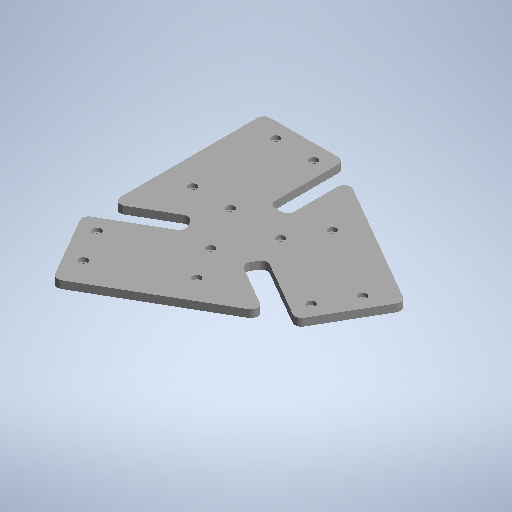
# Autodesk Inventor part: TestBench_Top_Motor_Support
Saved by Autodesk Inventor 2025.4 (Build 294407000, 407)
## iProperties
Created: 2026-05-15
Part Number: TestBench_Top_Motor_Support
Material: Générique
Document SubType Name: Modeling
Designer: louis
Density: 1 g/cm^3
Appearance: Par défaut
Author: louis
Autodesk Inventor part; units mm, degrees
ref_plane "YZ Plane" through (0, 0, 0) normal (1, 0, 0) x (0, 1, 0)
ref_plane "XZ Plane" through (0, 0, 0) normal (0, 1, 0) x (-1, 0, 0)
ref_plane "XY Plane" through (0, 0, 0) normal (0, 0, 1) x (1, 0, 0)
sketch "Sketch2" plane through (0, 0, 0) normal (0, 0, 1) x (1, 0, 0)
  line L0 (-50, 78) -> (-50, 12) construction
  line L1 (-50, 12) -> (-20, 12) construction
  line L2 (-20, 12) -> (-20, 78) construction
  line L3 (-20, 78) -> (-50, 78) construction
  line L4 (-50, 78) -> (-20, 12) construction
  line L5 (-50, 12) -> (-20, 78) construction
  line L6 (-7.5, 90) -> (7.5, 90)
  line L7 (7.5, 90) -> (7.5, 0)
  line L8 (7.5, 0) -> (-7.5, 0)
  line L9 (-7.5, 0) -> (-7.5, 90)
  line L10 (-7.5, 90) -> (7.5, 0) construction
  line L11 (7.5, 90) -> (-7.5, 0) construction
  line L12 (-35, 45) -> (0, 45) construction
  line L13 (0, 45) -> (0, 0) construction
  line L14 (-7.5, 30) -> (7.5, 30)
  line L15 (7.5, 30) -> (64.1758, 30)
  circle A0 centre (0, 0) radius 115 construction
  line L16 (0, 0) -> (0, 30)
  line L17 (0, 0) -> (-99.5929, -57.5)
  line L18 (-7.5, 90) -> (-7.5, 114.7552)
  line L19 (-71.5891, -41.332) -> (-71.5891, 90)
  line L20 (-71.5891, 90) -> (-7.5, 90)
  line L21 (-22.2308, -21.4952) -> (-29.7308, -8.5048)
  line L22 (-81.6923, -38.5048) -> (-3.75, 6.4952)
  line L23 (3.75, -6.4952) -> (-74.1923, -51.4952)
  line L24 (-74.1923, -51.4952) -> (-81.6923, -38.5048)
  line L25 (-3.75, 6.4952) -> (3.75, -6.4952)
  line L26 (29.7308, -8.5048) -> (22.2308, -21.4952)
  line L27 (74.1923, -51.4952) -> (-3.75, -6.4952)
  line L28 (3.75, 6.4952) -> (81.6923, -38.5048)
  line L29 (81.6923, -38.5048) -> (74.1923, -51.4952)
  line L30 (-3.75, -6.4952) -> (3.75, 6.4952)
  point P0 (-25.9808, -15)
  point P1 (25.9808, -15)
  point P2 (-71.5891, -32.6717)
  point P3 (-25.9808, -15)
  dimension "d0" = 30
  dimension "d1" = 66
  dimension "d2" = 15
  dimension "d3" = 90
  dimension "d4" = 12.5
  dimension "d5" = 45
  dimension "d6" = 30
  dimension "d15" = 120
  dimension "d16" = 115
  dimension "d31" = 360
  constraints: 62 end point, 7 point on line, 5 coincident, 5 midpoint, 4 parallel, 4 perpendicular, 4 vertical, 3 horizontal, 3 point on circle, 1 centre point, 37 other
  measures "d0" distance of L2.end L0.start
  measures "d1" distance of L1.end L2.end
  measures "d2" distance of L7.end L8.end
  measures "d3" distance of L6.end L7.end
  measures "d4" distance between parallel lines of L2 L9
  measures "d5" distance from line of L13.end L12
  measures "d6" distance from line of L14 L13.end
  measures "d15" angle of L13 L17
  measures "d16" distance of L16.start L17.end
extrude "Extrusion1" add sketch "Sketch2" against normal blind 6 contours L9 L22 L19 L20 | L14 L16 L25 L22 L9 | L22 L25 L8 L9 | L9 L8 L17 L21 L22
hole "Hole1" at (-50, 78, 0) at (-20, 78, 0) at (-20, 12, 0) at (-50, 12, 0) direction (0, 0, -1) diameter 3.6 end through all counterbore diameter 6.5 counterbore depth 3 clearance for "Socket Head Cap Screw" size "M3" standard "Ansi Metric M Profile"
pattern_circular "Circular Pattern1" count 3 over 360 about axis through (0, 0, 0) along (0, 0, -1) of "Extrusion1", "Hole1"
fillet "Fillet1" radius 5 15 edges at (113.7368, 16.998, -3) (81.6923, -38.5048, -3) (-7.5, 90, -3) (-71.5891, 90, -3) (-7.5, 30, -3) (-74.1923, -51.4952, -3) (-22.2308, -21.4952, -3) (-42.1477, -106.998, -3) (29.7308, -8.5048, -3) (7.5, 78.3339, -3) (7.5, 30, -3) (22.2308, -21.4952, -3) (-29.7308, -8.5048, -3) (64.0891, -45.6621, -3) (-71.5891, -32.6717, -3)
body "Solid1"
